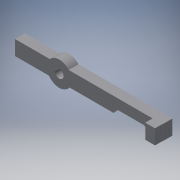
# Autodesk Inventor part: Reset_beam
Saved by Autodesk Inventor 2019.3 (Build 233278000, 278)
## iProperties
Created: 2020-10-09
Part Number: Reset_beam
Material: Generisch
Document SubType Name: Modeling
Designer: Nicolas Frick
Density: 1 g/cm^3
Appearance: Vorgabe
Author: Nicolas Frick
Autodesk Inventor part; units mm, degrees
ref_plane "YZ Plane" through (0, 0, 0) normal (1, 0, 0) x (0, 1, 0)
ref_plane "XZ Plane" through (0, 0, 0) normal (0, 1, 0) x (-1, 0, 0)
ref_plane "XY Plane" through (0, 0, 0) normal (0, 0, 1) x (1, 0, 0)
sketch "Skizze1" plane through (0, 0, 0) normal (0, 0, 1) x (1, 0, 0)
  line L0 (2, -8) -> (-6, -8) construction
  line L1 (2, 0) -> (2, -8) construction
  line L2 (0, 0) -> (2, 0) construction
  line L3 (0, 1.7577) -> (0, 0) construction
  line L4 (2, 1.7577) -> (0, 1.7577) construction
  line L5 (2, 1.7577) -> (2, 8.4467) construction
  line L6 (0, 8.4467) -> (2, 8.4467) construction
  line L7 (0, 11) -> (0, 8.4467) construction
  line L8 (-6, 11) -> (0, 11) construction
  line L9 (-6, -8) -> (-6, 11) construction
  circle A0 centre (-3, -3.7188) radius 1.75 construction
  circle A1 centre (-3, -3.7188) radius 1.75
  line L10 (5.65, 17) -> (8.35, 17) construction
  line L11 (11, -0.5) -> (11, 14.5) construction
  line L12 (3, -0.5) -> (11, -0.5) construction
  line L13 (3, -0.5) -> (3, 14.5) construction
  line L14 (7, 17) -> (39, 17) construction
  line L15 (0.8261, -0.5) -> (39, -0.5)
  line L16 (39, -0.5) -> (39, -6.5)
  line L17 (39, -6.5) -> (1.1551, -6.5)
  line L18 (-6.8261, -0.5) -> (-21, -0.5)
  line L19 (-21, -0.5) -> (-21, -6.5)
  line L20 (-21, -6.5) -> (-7.1551, -6.5)
  line L21 (-6, -6.5) -> (-6, -0.5) construction
  arc A2 (0.8261, -0.5) -> (-6.8261, -0.5) centre (-3, -3.7188) ccw
  arc A3 (-7.1551, -6.5) -> (1.1551, -6.5) centre (-3, -3.7188) ccw
  dimension "d0" = 32
  dimension "d1" = 6
  dimension "d2" = 15
  constraints: 20 end point, 4 point on circle, 3 centre point, 3 horizontal, 3 parallel, 3 point on line, 2 coincident, 2 perpendicular, 2 vertical, 1 concentric, 1 midpoint, 3 other
  measures "d0" distance of L14.start L14.end
  measures "d1" distance of L15.end L16.end
  measures "d2" distance of L21.start L19.end
extrude "Extrusion1" add sketch "Skizze1" along normal blind 4
sketch "Skizze2" plane through (1.1551, -6.5, 0) normal (0, -1, 0) x (1, 0, 0)
  line L0 (37.7621, 0) -> (33.7621, 0)
  line L1 (33.7621, 0) -> (33.7621, 7)
  line L2 (33.7621, 7) -> (37.7621, 7)
  line L3 (37.7621, 7) -> (37.7621, 0)
  point P0 (-1.1551, 0)
  dimension "d5" = 4
  dimension "d6" = 7
  constraints: 8 end point, 2 parallel, 1 horizontal, 1 perpendicular
  measures "d5" distance of L1.end L2.end
  measures "d6" distance of L0.end L1.end
extrude "Extrusion3" add sketch "Skizze2" against normal blind 6
sketch "Skizze3" plane through (0, 0, 4) normal (0, 0, 1) x (1, 0, 0)
  circle A0 centre (-3, -3.7188) radius 1.75 construction
  line L0 (34.9172, -6.5) -> (34.9172, -0.5) construction
  line L1 (34.9172, -0.5) -> (0.8261, -0.5) construction
  arc A1 (0.8261, -0.5) -> (-6.8261, -0.5) centre (-3, -3.7188) ccw construction
  line L2 (-6.8261, -0.5) -> (-21, -0.5) construction
  line L3 (-21, -0.5) -> (-21, -6.5) construction
  line L4 (-21, -6.5) -> (-7.1551, -6.5) construction
  arc A2 (-7.1551, -6.5) -> (1.1551, -6.5) centre (-3, -3.7188) ccw construction
  line L5 (1.1551, -6.5) -> (34.9172, -6.5) construction
  line L6 (34.9172, -4.4009) -> (29.9172, -4.4009) construction
  arc A3 (33.0892, -6.5) -> (19.0718, -6.5) centre (26.0805, -10.6676) ccw
  line L7 (19.0718, -6.5) -> (33.0892, -6.5)
  line L8 (1.1551, -6.5) -> (34.9172, -6.5) construction
  point P0 (0, 0)
  dimension "d11" = 5
  constraints: 4 end point, 4 point on line, 2 point on circle, 1 centre point, 1 horizontal
  measures "d11" distance of L6.start L6.end
extrude "Extrusion4" cut sketch "Skizze3" against normal blind 6
sketch "Skizze4" plane through (0, 0, 4) normal (0, 0, 1) x (1, 0, 0)
  arc A0 (33.0892, -6.5) -> (19.0718, -6.5) centre (26.0805, -10.6676) ccw construction
  line L0 (33.0892, -6.5) -> (34.9172, -6.5) construction
  line L1 (34.9172, -6.5) -> (34.9172, -0.5) construction
  line L2 (34.9172, -0.5) -> (0.8261, -0.5) construction
  arc A1 (0.8261, -0.5) -> (-6.8261, -0.5) centre (-3, -3.7188) ccw construction
  line L3 (-6.8261, -0.5) -> (-21, -0.5) construction
  line L4 (-21, -0.5) -> (-21, -6.5) construction
  line L5 (-21, -6.5) -> (-7.1551, -6.5) construction
  arc A2 (-7.1551, -6.5) -> (1.1551, -6.5) centre (-3, -3.7188) ccw construction
  line L6 (1.1551, -6.5) -> (19.0718, -6.5) construction
  circle A3 centre (-3, -3.7188) radius 1.75 construction
  line L7 (17.8717, -0.5) -> (33.0892, -0.5)
  line L8 (33.0892, -0.5) -> (33.0892, -4.6064)
  line L9 (33.0892, -4.6064) -> (17.8717, -4.6064)
  line L10 (17.8717, -4.6064) -> (17.8717, -0.5)
  point P0 (0, 0)
  constraints: 8 end point, 2 parallel, 1 horizontal, 1 midpoint, 1 perpendicular
extrude "Extrusion5" add sketch "Skizze4" against normal blind 4
